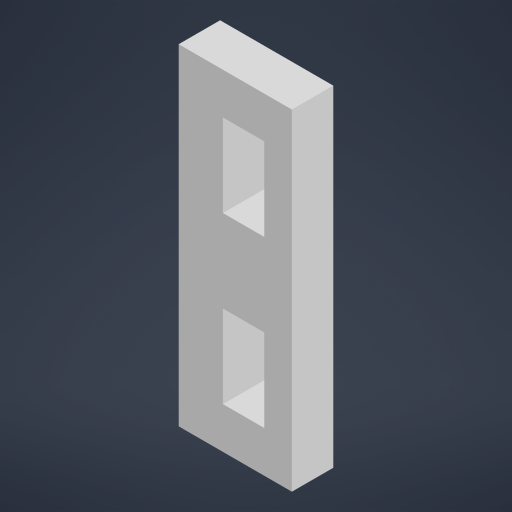
# Autodesk Inventor part: SideClip
Saved by Autodesk Inventor 2023 (Build 270158000, 158)
## iProperties
Created: 2023-03-14
Part Number: SideClip
Material: Generic
Document SubType Name: Modeling
Designer: Matt
Density: 1 g/cm^3
Appearance: Default
Author: Matt
Autodesk Inventor part; units mm, degrees
ref_plane "YZ Plane" through (0, 0, 0) normal (1, 0, 0) x (0, 1, 0)
ref_plane "XZ Plane" through (0, 0, 0) normal (0, 1, 0) x (-1, 0, 0)
ref_plane "XY Plane" through (0, 0, 0) normal (0, 0, 1) x (1, 0, 0)
sketch "Sketch1" plane through (0, 0, 0) normal (0, 0, 1) x (1, 0, 0)
  line L0 (0, 0) -> (8.2022, 0)
  line L1 (8.2022, 0) -> (8.2022, 24)
  line L2 (8.2022, 24) -> (0, 24)
  line L3 (0, 24) -> (0, 0)
  line L4 (6.2022, 21) -> (3.2022, 21)
  line L5 (3.2022, 21) -> (3.2022, 15)
  line L6 (3.2022, 15) -> (6.2022, 15)
  line L7 (6.2022, 15) -> (6.2022, 21)
  line L8 (10.1659, 12) -> (-5.2678, 12)
  line L9 (6.2022, 3) -> (3.2022, 3)
  line L10 (3.2022, 3) -> (3.2022, 9)
  line L11 (3.2022, 9) -> (6.2022, 9)
  line L12 (6.2022, 9) -> (6.2022, 3)
  dimension "d0" = 24
  dimension "d1" = 3
  dimension "d2" = 6
  dimension "d3" = 3
  dimension "d4" = 2
  constraints: 26 end point, 4 parallel, 4 symmetric about line, 3 horizontal, 2 perpendicular
  measures "d0" distance of L0.end L1.end
  measures "d1" distance of L4.start L4.end
  measures "d2" distance of L6.end L4.start
  measures "d3" distance between parallel lines of L2 L4
  measures "d4" distance between parallel lines of L1 L7
extrude "Extrusion1" add sketch "Sketch1" along normal blind 3
equation "\"d0\" = CameraHeight"
equation "\"d1\" = Acrylic"
equation "\"d2\" = 0.25 * CameraHeight"
equation "\"d5\" = Acrylic"
equation "\"Acrylic\" = 3"
equation "\"CameraHeight\" = 24"
equation "\"CameraWidth\" = 25"
body "Solid1"
